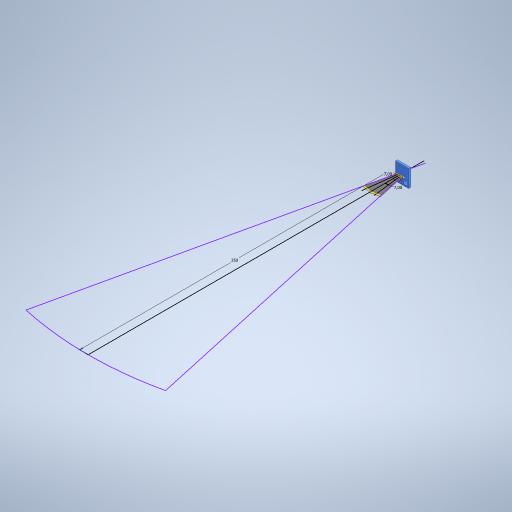
# Autodesk Inventor part: TOF_VLCOS
Saved by Autodesk Inventor 2023 (Build 270158000, 158)
## iProperties
Created: 2022-12-13
Part Number: TOF_VLCOS
Material: Generic
Document SubType Name: Modeling
Designer: Kamil
Density: 1 g/cm^3
Appearance: Default
Author: Kamil
Autodesk Inventor part; units mm, degrees
ref_plane "YZ Plane" through (0, 0, 0) normal (1, 0, 0) x (0, 1, 0)
ref_plane "XZ Plane" through (0, 0, 0) normal (0, 1, 0) x (-1, 0, 0)
ref_plane "XY Plane" through (0, 0, 0) normal (0, 0, 1) x (1, 0, 0)
sketch "Sketch1" plane through (0, 0, 0) normal (0, 0, 1) x (1, 0, 0)
  line L0 (-6.698639, 7.691729) -> (4.001361, 7.691729)
  line L1 (4.001361, 7.691729) -> (4.001361, -6.308271)
  line L2 (4.001361, -6.308271) -> (-6.698639, -6.308271)
  line L3 (-6.698639, -6.308271) -> (-6.698639, 7.691729)
  line L4 (4.001361, -6.308271) -> (-6.698639, -6.308271)
  line L5 (-6.698639, -6.308271) -> (-6.698639, -2.808271)
  line L6 (-6.698639, -2.808271) -> (4.001361, -2.808271)
  line L7 (4.001361, -2.808271) -> (4.001361, -6.308271)
  line L8 (-6.698639, -6.308271) -> (-5.698639, -6.308271)
  line L9 (-5.698639, -6.308271) -> (-5.698639, 7.691729)
  line L10 (-5.698639, 7.691729) -> (-6.698639, 7.691729)
  line L11 (-6.698639, 7.691729) -> (-6.698639, -6.308271)
  line L12 (-5.698639, -2.808271) -> (3.472299, -2.808271)
  line L13 (3.472299, -2.808271) -> (3.472299, -0.408271)
  line L14 (3.472299, -0.408271) -> (-5.698639, -0.408271)
  line L15 (-5.698639, -0.408271) -> (-5.698639, -2.808271)
  line L16 (-5.698639, -0.408271) -> (-1.298639, -0.408271)
  line L17 (-1.298639, -0.408271) -> (-1.298639, -2.808271)
  line L18 (-1.298639, -2.808271) -> (-5.698639, -2.808271)
  line L19 (-5.698639, -2.808271) -> (-5.698639, -0.408271)
  point P0 (0, 0)
  dimension "d0" = 10.7
  dimension "d1" = 14
  dimension "d2" = 3.5
  dimension "d3" = 1
  dimension "d4" = 2.4
  dimension "d5" = 4.4
  constraints: 40 end point, 10 parallel, 5 horizontal, 5 perpendicular, 5 point on line
  measures "d0" distance of L1.end L2.end
  measures "d1" distance of L0.end L1.end
  measures "d2" distance of L4.end L5.end
  measures "d3" distance of L10.end L9.end
  measures "d4" distance of L13.end L12.end
  measures "d5" distance of L17.end L18.end
extrude "Extrusion1" add sketch "Sketch1" against normal blind 1.6
extrude "Extrusion2" add sketch "Sketch1" along normal blind 1.1 contours L14 L17 L6 L9
sketch "Sketch2" plane through (0, 0, 0) normal (0, 0, 1) x (1, 0, 0)
  line L0 (-1.298639, -0.408271) -> (-1.298639, -2.808271)
  line L1 (-1.298639, -2.808271) -> (-5.698639, -2.808271)
  line L2 (-5.698639, -2.808271) -> (-5.698639, -0.408271)
  line L3 (-5.698639, -0.408271) -> (-1.298639, -0.408271)
  line L4 (4.001361, 7.691729) -> (-6.698639, 7.691729)
  line L5 (-6.698639, 7.691729) -> (-6.698639, -6.308271)
  line L6 (-6.698639, -6.308271) -> (4.001361, -6.308271)
  line L7 (4.001361, -6.308271) -> (4.001361, 7.691729)
  line L8 (4.001361, -6.308271) -> (4.001361, 7.691729)
  line L9 (-6.698639, 7.691729) -> (-6.698639, -6.308271)
  line L10 (4.001361, -6.308271) -> (-6.698639, -6.308271)
  line L11 (-6.698639, -6.308271) -> (-6.698639, -5.308271)
  line L12 (-6.698639, -5.308271) -> (4.001361, -5.308271)
  line L13 (4.001361, -5.308271) -> (4.001361, -6.308271)
  line L14 (4.001361, -6.308271) -> (3.001361, -6.308271)
  line L15 (3.001361, -6.308271) -> (3.001361, -2.808271)
  line L16 (3.001361, -2.808271) -> (4.001361, -2.808271)
  line L17 (4.001361, -2.808271) -> (4.001361, -6.308271)
  line L18 (-6.698639, -6.308271) -> (-0.098639, -6.308271)
  line L19 (-0.098639, -6.308271) -> (-0.098639, -2.808271)
  line L20 (-0.098639, -2.808271) -> (-6.698639, -2.808271)
  line L21 (-6.698639, -2.808271) -> (-6.698639, -6.308271)
  circle A0 centre (1.451361, -3.758271) radius 1.55
  point P0 (0, 0)
  dimension "d10" = 1
  dimension "d11" = 1
  dimension "d12" = 6.6
  constraints: 24 end point, 6 parallel, 3 horizontal, 3 perpendicular, 3 tangent, 1 centre point, 1 point on line
  measures "d10" distance of L10.end L11.end
  measures "d11" distance of L15.end L16.end
  measures "d12" distance of L20.end L19.end
extrude "Extrusion3" cut sketch "Sketch2" against normal through all contours A0
sketch "Sketch3" plane through (0, 0, 0) normal (0, 0, 1) x (1, 0, 0)
  line L0 (4.001361, 7.691729) -> (4.001361, -6.308271)
  line L1 (-6.698639, 7.691729) -> (4.001361, 7.691729)
  line L2 (4.001361, 7.691729) -> (4.001361, 6.691729)
  line L3 (4.001361, 6.691729) -> (-6.698639, 6.691729)
  line L4 (-6.698639, 6.691729) -> (-6.698639, 7.691729)
  line L5 (-6.698639, 7.691729) -> (-5.698639, 7.691729)
  line L6 (-5.698639, 7.691729) -> (-5.698639, 5.612457)
  line L7 (-5.698639, 5.612457) -> (-6.698639, 5.612457)
  line L8 (-6.698639, 5.612457) -> (-6.698639, 7.691729)
  line L9 (-5.698639, 6.691729) -> (-4.598639, 6.691729)
  line L10 (-4.598639, 6.691729) -> (-4.598639, 6.161753)
  line L11 (-4.598639, 6.161753) -> (-5.698639, 6.161753)
  line L12 (-5.698639, 6.161753) -> (-5.698639, 6.691729)
  circle A0 centre (-5.148639, 6.141729) radius 0.55
  circle A1 centre (-2.608639, 6.141729) radius 0.55
  line L13 (-2.058639, 6.161753) -> (-3.158639, 6.161753)
  circle A2 centre (-0.068639, 6.141729) radius 0.55
  line L14 (0.481361, 6.161753) -> (-0.618639, 6.161753)
  circle A3 centre (2.471361, 6.141729) radius 0.55
  line L15 (3.021361, 6.161753) -> (1.921361, 6.161753)
  circle A4 centre (1.451361, -3.758271) radius 1.55
  line L16 (-1.298639, -0.408271) -> (-1.298639, -2.808271)
  line L17 (-1.298639, -2.808271) -> (-5.698639, -2.808271)
  line L18 (-5.698639, -2.808271) -> (-5.698639, -0.408271)
  line L19 (-5.698639, -0.408271) -> (-1.298639, -0.408271)
  line L20 (4.001361, 7.691729) -> (-6.698639, 7.691729)
  line L21 (-6.698639, 7.691729) -> (-6.698639, -6.308271)
  line L22 (-6.698639, -6.308271) -> (4.001361, -6.308271)
  line L23 (4.001361, -6.308271) -> (4.001361, 7.691729)
  line L24 (-6.698639, -6.308271) -> (-5.698639, -6.308271)
  line L25 (-5.698639, -6.308271) -> (-5.698639, -3.371834)
  line L26 (-5.698639, -3.371834) -> (-6.698639, -3.371834)
  line L27 (-6.698639, -3.371834) -> (-6.698639, -6.308271)
  line L28 (-6.698639, -6.308271) -> (4.001361, -6.308271)
  line L29 (-6.698639, -6.308271) -> (-3.498639, -6.308271)
  line L30 (-3.498639, -6.308271) -> (-3.498639, -5.308271)
  line L31 (-3.498639, -5.308271) -> (-6.698639, -5.308271)
  line L32 (-6.698639, -5.308271) -> (-6.698639, -6.308271)
  line L33 (-5.698639, -6.308271) -> (-4.598639, -6.308271)
  line L34 (-4.598639, -6.308271) -> (-4.598639, -3.371834)
  line L35 (-4.598639, -3.371834) -> (-5.698639, -3.371834)
  line L36 (-5.698639, -3.371834) -> (-5.698639, -6.308271)
  circle A5 centre (-5.148639, -4.758271) radius 0.55
  circle A6 centre (-2.608639, -4.758271) radius 0.55
  line L37 (-0.958639, -5.308271) -> (-4.158639, -5.308271)
  point P0 (0, 0)
  dimension "d15" = 1
  dimension "d16" = 1
  dimension "d17" = 1.1
  dimension "d20" = 2.54
  dimension "d25" = 1
  dimension "d26" = 1
  dimension "d27" = 1.1
  dimension "d30" = 2.54
  constraints: 56 end point, 12 parallel, 8 horizontal, 6 centre point, 6 perpendicular, 6 tangent, 4 point on line, 2 collinear, 18 other
  measures "d15" distance of L1.end L2.end
  measures "d16" distance of L6.end L7.end
  measures "d17" distance of L10.end L11.end
  measures "d20" distance of A0.centre A1.centre
  measures "d25" distance of L26.end L25.end
  measures "d26" distance of L30.end L29.end
  measures "d27" distance of L35.end L34.end
  measures "d30" distance of A5.centre A6.centre
sketch "Sketch3 outline for Extrusion4" plane through (0, 0, 0) normal (0, 0, 1) x (1, 0, 0)
  circle A0 centre (-5.148639, -4.758271) radius 0.55
  circle A1 centre (-2.608639, -4.758271) radius 0.55
  circle A2 centre (2.471361, 6.141729) radius 0.55
  circle A3 centre (-0.068639, 6.141729) radius 0.55
  circle A4 centre (-2.608639, 6.141729) radius 0.55
  circle A5 centre (-5.148639, 6.141729) radius 0.55
extrude "Extrusion4" cut sketch "Sketch3 outline for Extrusion4" against normal through all
sketch "Sketch4" plane through (-5.698639, -0.408271, 0) normal (0, 1, 0) x (1, 0, 0)
  line L0 (0, 0) -> (4.4, 0)
  line L1 (0, 0) -> (0, -1.1)
  line L2 (4.4, -1.1) -> (0, -1.1)
  line L3 (4.4, 0) -> (4.4, -1.1)
  line L4 (0, -1.1) -> (-17.024616, -77.893079)
  line L5 (4.4, -1.1) -> (11.53177, -33.269335)
  line L6 (2.2, -1.1) -> (2.2, -23.383849)
  line L7 (4.4, -1.1) -> (0, -1.1)
  line L8 (11.53177, -33.269335) -> (26.881941, -102.509481)
  circle A0 centre (2.2, -1.1) radius 22.283849
  line L9 (2.2, -23.383849) -> (9.005719, -21.875057)
  line L10 (2.2, -23.383849) -> (-4.605719, -21.875057)
  point P0 (5.698639, 0)
  dimension "d37" = 12.5
  dimension "d38" = 12.5
  constraints: 12 end point, 3 perpendicular, 2 point on line, 1 coincident, 1 collinear, 1 midpoint, 1 vertical alignment, 2 other
  measures "d37" angle of L6 L5
  measures "d38" angle of L4 L6
extrude "Wyciągnięcie proste5" add sketch "Sketch4" against normal blind 1 contours L2 L6 L10 L4 | L5 L9 L6 L2
sketch "Szkic5" plane through (-5.698639, -0.408271, 0) normal (0, 1, 0) x (1, 0, 0)
  line L0 (0, 0) -> (4.4, 0)
  line L1 (0, 0) -> (0, -1.1)
  line L2 (0, -1.1) -> (-4.605719, -21.875057)
  line L3 (-4.605719, -21.875057) -> (2.2, -23.383849)
  line L4 (2.2, -23.383849) -> (9.005719, -21.875057)
  line L5 (9.005719, -21.875057) -> (4.4, -1.1)
  line L6 (4.4, 0) -> (4.4, -1.1)
  line L7 (0, -1.1) -> (4.4, -1.1)
  line L8 (4.4, -1.1) -> (26.847507, -102.354162)
  line L9 (2.2, -1.1) -> (2.2, -251.1)
  line L10 (26.847507, -102.354162) -> (58.457755, -244.938774)
  line L11 (0, -1.1) -> (-54.057755, -244.938774)
  line L12 (2.2, -1.1) -> (2.2, 19.845326)
  line L13 (0, -1.1) -> (4.4, 18.747117)
  arc A0 (-54.057755, -244.938774) -> (58.457755, -244.938774) centre (2.2, 8.823559) ccw
  line L14 (2.2, -251.1) -> (0, -251.1)
  point P0 (5.698639, 0)
  dimension "d41" = 250
  constraints: 14 end point, 3 point on circle, 2 midpoint, 2 vertical, 1 centre point, 1 horizontal, 1 point on line
  measures "d41" distance of L9.start L9.end
sketch "Szkic6" plane through (-5.698639, -0.408271, 0) normal (0, 1, 0) x (1, 0, 0)
  line L0 (2.2, -23.383849) -> (-4.605719, -21.875057)
  line L1 (-4.605719, -21.875057) -> (2.53543, 10.336584)
  line L2 (9.005719, -21.875057) -> (2.2, -23.383849)
  line L3 (9.005719, -21.875057) -> (2.2, 8.823559)
  line L4 (2.2, 8.823559) -> (2.2, -23.383849)
  line L5 (2.2, 8.823559) -> (-2.082149, -26.051744)
  line L6 (2.2, 8.823559) -> (6.293179, -24.512711)
  point P0 (5.698639, 0)
  dimension "d42" = 7
  dimension "d43" = 7
  constraints: 10 end point, 1 perpendicular, 1 point on line, 1 vertical
  measures "d42" angle of L4 L6
  measures "d43" angle of L4 L5
body "Solid1"
